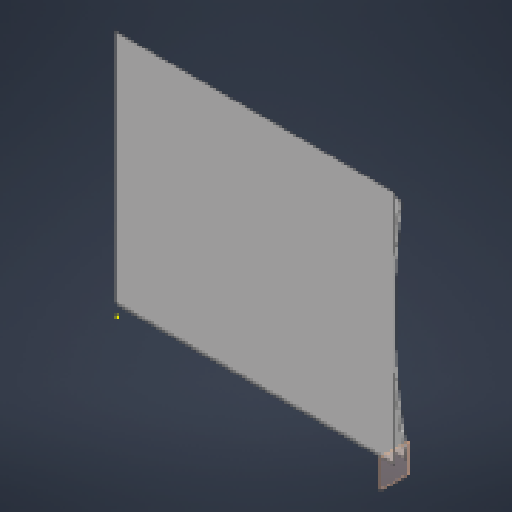
# Autodesk Inventor part: наклон
Saved by Autodesk Inventor 2025 (Build 290162000, 162)
## iProperties
Created: 2025-09-06
Part Number: наклон
Material: Типовые
Document SubType Name: Modeling
Designer: Trene
Density: 1 g/cm^3
Appearance: По умолчанию
Author: Trene
Autodesk Inventor part; units mm, degrees
ref_plane "YZ Plane" through (0, 0, 0) normal (1, 0, 0) x (0, 1, 0)
ref_plane "XZ Plane" through (0, 0, 0) normal (0, 1, 0) x (-1, 0, 0)
ref_plane "XY Plane" through (0, 0, 0) normal (0, 0, 1) x (1, 0, 0)
sketch "Эскиз1" plane through (0, 0, 0) normal (0, 0, 1) x (1, 0, 0)
  line L0 (0, 0) -> (130, 0)
  line L1 (130, 0) -> (130, 240)
  line L2 (130, 240) -> (0, 240)
  line L3 (0, 240) -> (0, 0)
  dimension "d0" = 130
  dimension "d1" = 240
  constraints: 8 end point, 2 parallel, 1 horizontal, 1 perpendicular
  measures "d0" distance of L2.end L1.end
  measures "d1" distance of L1.end L0.end
extrude "Выдавливание1" add sketch "Эскиз1" along normal blind 1.5
ref_plane "РабПлоскость1" through (130, 7.8819, 0) normal (1, 0, 0) x (0, 0, -1)
sketch "Эскиз3" plane through (130, 7.8819, 0) normal (1, 0, 0) x (0, 0, -1)
  line L0 (-1.5, 2.8482) -> (0, 0) projected
  line L1 (0, 0) -> (-1.5, 2.8482)
  line L2 (0, -7.8819) -> (0, 232.1181) projected
  line L3 (0, 232.1181) -> (-1.5, 232.1181) projected
  line L4 (-1.5, -7.8819) -> (-1.5, 232.1181) projected
  line L5 (0, -7.8819) -> (-1.5, -7.8819) projected
  point P0 (0, -7.8819)
  point P1 (0, 0)
  point P2 (-1.5, 2.8482)
  constraints: 2 end point, 1 collinear
extrude "Выдавливание3" cut sketch "Эскиз3" against normal through all contours L0 L2 L5 L4
sketch "Эскиз4" plane through (0, 0, 0) normal (0, 0, -1) x (-1, 0, 0)
  line L0 (-186.9271, 194.527) -> (57.0729, 194.527) projected
  line L1 (-130, 7.8819) -> (0, 7.8819) projected
  line L2 (0, 240) -> (0, 7.8819) projected
  line L3 (-130, 240) -> (0, 240) projected
  line L4 (-130, 7.8819) -> (-130, 240) projected
  point P0 (0, 0)
  point P1 (-130, 194.527)
  point P2 (0, 194.527)
extrude "Выдавливание4" cut sketch "Эскиз4" against normal blind 10 contours L4 L3 L2 L0
sketch "Эскиз5" plane through (0, 7.8819, 0) normal (-1, 0, 0) x (0, 0, 1)
  line L0 (1.5, 186.6451) -> (0, 186.6451) projected
  line L1 (0, 186.6451) -> (0, 0) projected
  line L2 (0, 0) -> (1.5, 2.8482) projected
  line L3 (1.5, 186.6451) -> (1.5, 2.8482) projected
  point P0 (0, -7.8819)
extrude "Выдавливание5" add sketch "Эскиз5" along normal blind 84
sketch "Эскиз6" plane through (130, 7.8819, 0) normal (1, 0, 0) x (0, 0, -1)
  line L0 (0, 186.6451) -> (0, 0) projected
  line L1 (0, 0) -> (-1.5, 2.8482) projected
  line L2 (-1.5, 2.8482) -> (-1.5, 186.6451) projected
  line L3 (-1.5, 186.6451) -> (0, 186.6451) projected
  line L4 (8.5, 202.2968) -> (8.5, 0)
  circle A0 centre (515.0502, 101.1484) radius 516.5502
  circle A1 centre (515.0502, 101.1484) radius 514.5502
  point P0 (0, -7.8819)
  point P1 (8.5, 10.767)
  point P2 (8.5, 191.5298)
  point P3 (0, 140.4854)
  point P4 (0, 61.8114)
  dimension "d14" = 10
  dimension "d15" = 2
  constraints: 2 centre point, 2 end point, 2 point on circle, 1 tangent, 1 vertical
  measures "d14" distance between parallel lines of L2 L4
  measures "d15" radial gap between concentric circles of A0 A1
extrude "Выдавливание6" add sketch "Эскиз6" against normal up to surface (214 mm away) contours A0 L4 A1 L0
sketch "Эскиз7" plane through (-84, 7.8819, 0) normal (-1, 0, 0) x (0, 0, 1)
  point P0 (0, -7.8819)
sketch "Эскиз8" plane through (130, 10.73, 1.5) normal (1, 0, 0) x (0, 0, -1)
  line L0 (79.5151, 63.8331) -> (-133.933, 378.2212) projected
  line L1 (-7.5015, 192) -> (20.3347, 151)
  line L2 (20.3347, 151) -> (38.1037, 163.064)
  line L3 (38.1037, 163.064) -> (10.2675, 204.064)
  line L4 (10.2675, 204.064) -> (-7.5015, 192)
  point P0 (1.5, -10.73)
  constraints: 8 end point, 2 parallel, 2 point on line, 1 perpendicular
extrude "Выдавливание7" cut sketch "Эскиз8" against normal through all
